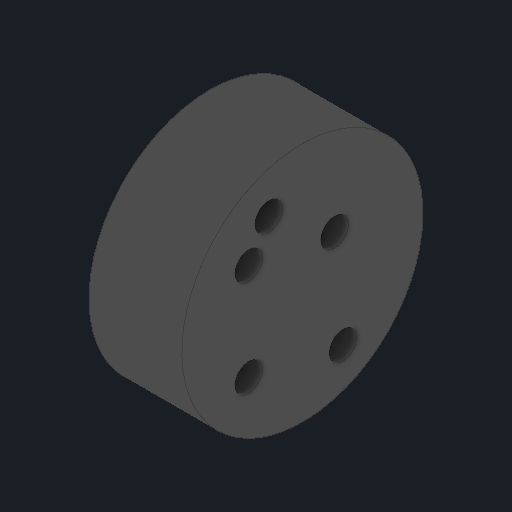
# Autodesk Inventor part: madeinlinux
Saved by Autodesk Inventor 2026 (Build 300175050, 175E)
## iProperties
Appearance: Default
Density: 1 g/cm^3
Designer: lachlan
Document SubType Name: Modeling
Material: Generic
Part Number: madeinlinux
Created: 2026-03-20
Author: lachlan
Autodesk Inventor part; units mm, degrees
ref_plane "YZ Plane" through (0, 0, 0) normal (1, 0, 0) x (0, 1, 0)
ref_plane "XZ Plane" through (0, 0, 0) normal (0, 1, 0) x (-1, 0, 0)
ref_plane "XY Plane" through (0, 0, 0) normal (0, 0, 1) x (1, 0, 0)
sketch "Sketch1" plane through (0, 0, 0) normal (1, 0, 0) x (0, 1, 0)
  circle A0 centre (0, 0) radius 12.9812
  constraints: 1 centre point, 1 coincident
extrude "Extrusion1" add sketch "Sketch1" along normal blind 10
sketch "Sketch2" plane through (10, 0, 0) normal (1, 0, 0) x (0, 0, -1)
  point P0 (0, 0)
  point P1 (3.4567, 2.9986)
  point P2 (-5.789, 4.4979)
  point P3 (-3.6233, 7.9963)
  point P4 (4.373, -7.9963)
  point P5 (-5.789, -5.9139)
hole "Hole1" at (10, 2.9986, -3.4567) at (10, 4.4979, 5.789) at (10, 7.9963, 3.6233) at (10, -7.9963, -4.373) at (10, -5.9139, 5.789) direction (-1, 0, 0) diameter 3 end through all
body "Solid1"
